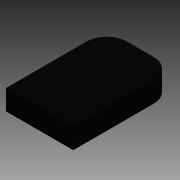
# Autodesk Inventor part: Fixture_Airpot_Support_2
Saved by Autodesk Inventor 2015 (Build 190159000, 159)
## iProperties
Created: 2014-12-16
Part Number: Fixture_Airpot_Support_2
Material: Generic
Document SubType Name: Modeling
Designer: amarschn
Density: 1 g/cm^3
Appearance: Anodized - Black
Author: amarschn
Autodesk Inventor part; units mm, degrees
ref_plane "YZ Plane" through (0, 0, 0) normal (1, 0, 0) x (0, 1, 0)
ref_plane "XZ Plane" through (0, 0, 0) normal (0, 1, 0) x (-1, 0, 0)
ref_plane "XY Plane" through (0, 0, 0) normal (0, 0, 1) x (1, 0, 0)
sketch "Sketch1" plane through (0, 0, 0) normal (0, 1, 0) x (-1, 0, 0)
  line L0 (-8.255, -31.4325) -> (8.255, -31.4325)
  line L1 (20.955, -18.7325) -> (20.955, 31.4325)
  line L2 (20.955, 31.4325) -> (-20.955, 31.4325)
  line L3 (-20.955, 31.4325) -> (-20.955, -18.7325)
  line L4 (-20.955, -31.4325) -> (20.955, 31.4325) construction
  line L5 (20.955, -31.4325) -> (-20.955, 31.4325) construction
  arc A0 (8.255, -31.4325) -> (20.955, -18.7325) centre (8.255, -18.7325) ccw
  arc A1 (-20.955, -18.7325) -> (-8.255, -31.4325) centre (-8.255, -18.7325) ccw
  point P0 (0, 0)
  dimension "d0" = 62.865
  dimension "d1" = 41.91
  dimension "d2" = 12.7
  constraints: 12 end point, 4 point on circle, 4 point on line, 4 tangent, 2 centre point, 2 midpoint, 2 parallel, 1 equal radius, 1 horizontal, 1 perpendicular
  measures "d0" distance of L5.start L1.end
  measures "d1" distance of L1.end L2.end
  measures "d2" radius of A0
extrude "Extrusion1" add sketch "Sketch1" along normal blind 12.7
body "Solid1"
